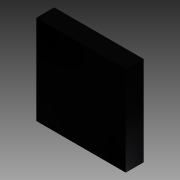
# Autodesk Inventor part: RFSwitch
Saved by Autodesk Inventor 2014 (Build 180170000, 170)
## iProperties
Created: 2015-03-25
Part Number: RFSwitch
Material: Generic
Document SubType Name: Modeling
Designer: Owner
Density: 1 g/cm^3
Appearance: Black
Author: Owner
Autodesk Inventor part; units mm, degrees
ref_plane "YZ Plane" through (0, 0, 0) normal (1, 0, 0) x (0, 1, 0)
ref_plane "XZ Plane" through (0, 0, 0) normal (0, 1, 0) x (-1, 0, 0)
ref_plane "XY Plane" through (0, 0, 0) normal (0, 0, 1) x (1, 0, 0)
sketch "Sketch1" plane through (0, 0, 0) normal (0, 0, 1) x (1, 0, 0)
  line L0 (-1.8474, 1.5158) -> (2.6526, 1.5158)
  line L1 (2.6526, 1.5158) -> (2.6526, -2.9842)
  line L2 (2.6526, -2.9842) -> (-1.8474, -2.9842)
  line L3 (-1.8474, -2.9842) -> (-1.8474, 1.5158)
  point P0 (0, 0)
  dimension "d0" = 4.5
  dimension "d1" = 4.5
  constraints: 8 end point, 2 parallel, 1 horizontal, 1 perpendicular
  measures "d0" distance of L0.start L0.end
  measures "d1" distance of L0.end L1.end
extrude "Extrusion1" add sketch "Sketch1" along normal blind 0.9
body "Solid1"
